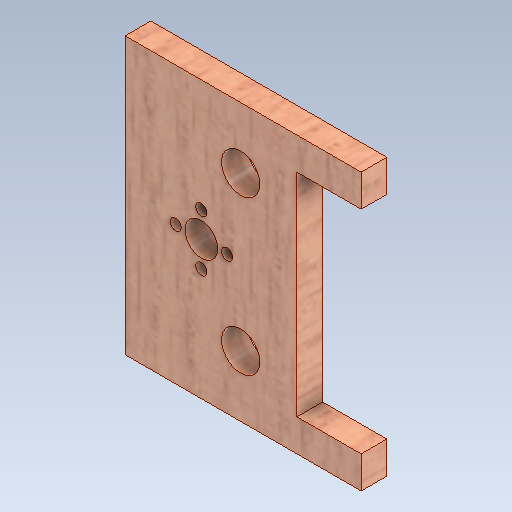
# Autodesk Inventor part: 0005-10-010
Saved by Autodesk Inventor 2020 (Build 240168000, 168)
## iProperties
Created: 2020-12-18
Part Number: 0005-10-010
Material: Generic
Document SubType Name: Modeling
Designer: Iulian Bors
Density: 1 g/cm^3
Appearance: White Oak - Natural Medium Gloss
Author: Iulian Bors
Subject: 010
Autodesk Inventor part; units mm, degrees
ref_plane "YZ Plane" through (0, 0, 0) normal (1, 0, 0) x (0, 1, 0)
ref_plane "XZ Plane" through (0, 0, 0) normal (0, 1, 0) x (-1, 0, 0)
ref_plane "XY Plane" through (0, 0, 0) normal (0, 0, 1) x (1, 0, 0)
sketch "Sketch1" plane through (0, 0, 0) normal (0, 0, 1) x (1, 0, 0)
  line L0 (-36.75, 43) -> (36.75, 43)
  line L1 (36.75, 43) -> (36.75, -43)
  line L2 (36.75, -43) -> (-36.75, -43)
  line L3 (-36.75, -43) -> (-36.75, 43)
  point P0 (0, 0)
  point P1 (0, 43)
  point P2 (-36.75, 0)
  dimension "d0" = 73.5
  dimension "d1" = 86
  constraints: 8 end point, 2 midpoint, 2 parallel, 1 horizontal, 1 horizontal alignment, 1 perpendicular, 1 vertical alignment
  measures "d0" distance of L0.start L0.end
  measures "d1" distance of L2.end L0.start
extrude "Extrusion1" add sketch "Sketch1" along normal blind 8
sketch "Sketch4" plane through (0, 0, 0) normal (0, 0, -1) x (-1, 0, 0)
  line L0 (-36.75, -33) -> (-16.75, -33)
  line L1 (-16.75, -33) -> (-16.75, 33)
  line L2 (-16.75, 33) -> (-36.75, 33)
  line L3 (-36.75, 33) -> (-36.75, -33)
  line L4 (-36.75, -43) -> (-36.75, 43) projected
  point P0 (0, 0)
  point P1 (-36.75, 0)
  dimension "d19" = 20
  dimension "d20" = 66
  constraints: 8 end point, 2 parallel, 1 collinear, 1 horizontal, 1 horizontal alignment, 1 midpoint, 1 perpendicular
  measures "d19" distance of L0.start L0.end
  measures "d20" distance of L0.end L1.end
extrude "Extrusion4" cut sketch "Sketch4" against normal blind 10
sketch "Sketch5" plane through (0, 0, 0) normal (0, 0, -1) x (-1, 0, 0)
  circle A0 centre (0.75, -24) radius 6
  circle A1 centre (0.75, 24) radius 6
  line L0 (-8.75, -33) -> (-8.75, 33) projected
  line L1 (-36.75, 33) -> (-36.75, 43) projected
  line L2 (-36.75, 43) -> (36.75, 43) projected
  line L3 (36.75, -43) -> (-36.75, -43) projected
  dimension "d23" = 12
  dimension "d37" = 37.5
  dimension "d38" = 19
  dimension "d39" = 19
  constraints: 2 centre point, 1 equal radius, 1 vertical alignment
  measures "d23" diameter of A0
  measures "d37" distance from line of L1 A1.centre
  measures "d38" distance from line of L2 A1.centre
  measures "d39" distance from line of L3 A0.centre
extrude "Extrusion5" cut sketch "Sketch5" against normal blind 10
sketch "Sketch6" plane through (0, 0, 0) normal (0, 0, -1) x (-1, 0, 0)
  circle A0 centre (12.9988, 0) radius 11
  circle A1 centre (12.9988, -8) radius 1.75
  circle A2 centre (4.9988, 0) radius 1.75
  circle A3 centre (12.9988, 8) radius 1.75
  circle A4 centre (20.9988, 0) radius 1.75
  circle A5 centre (12.9988, 0) radius 5.1
  circle A6 centre (12.9988, 0) radius 8 construction
  line L0 (36.75, 43) -> (36.75, -43) construction
  line L1 (-36.75, 43) -> (36.75, 43) construction
  point P0 (0, 0)
  dimension "d42" = 3.5
  dimension "d43" = 10.2
  dimension "d44" = 23.7512
  dimension "d46" = 22
  dimension "d47" = 16
  constraints: 7 centre point, 4 point on circle, 3 equal radius, 3 horizontal alignment, 2 vertical alignment, 1 coincident, 1 concentric
  measures "d42" diameter of A3
  measures "d43" diameter of A5
  measures "d44" distance from line of A5.centre L0
  measures "d46" diameter of A0
  measures "d47" diameter of A6
extrude "Extrusion6" cut sketch "Sketch6" against normal blind 10 contours A1 | A2 | A3 | A4 | A5
equation "\"d39\" = d38"
body "Solid1"
